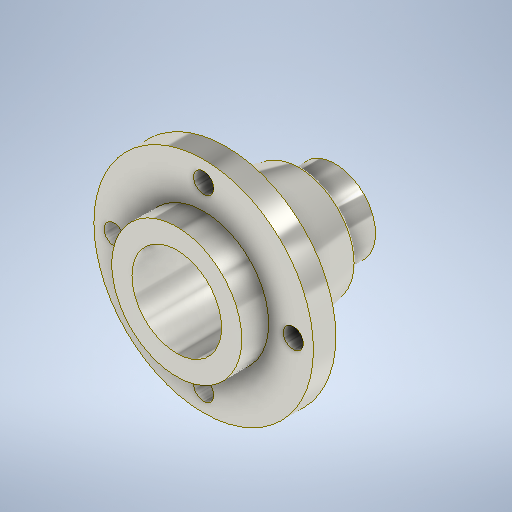
# Autodesk Inventor part: pokrywa
Saved by Autodesk Inventor 2025.2 (Build 292293000, 293)
## iProperties
Created: 2025-03-22
Part Number: pokrywa
Material: Srebro
Document SubType Name: Modeling
Designer: barte
Density: 10.49 g/cm^3
Appearance: Srebro
Author: barte
Autodesk Inventor part; units mm, degrees
ref_plane "YZ Plane" through (0, 0, 0) normal (1, 0, 0) x (0, 1, 0)
ref_plane "XZ Plane" through (0, 0, 0) normal (0, 1, 0) x (-1, 0, 0)
ref_plane "XY Plane" through (0, 0, 0) normal (0, 0, 1) x (1, 0, 0)
sketch "Szkic1" plane through (0, 0, 0) normal (0, 1, 0) x (-1, 0, 0)
  line L0 (34.3124, 12.606) -> (49, 12.606)
  line L1 (0, 12.606) -> (0, -21.394)
  line L2 (20, -21.394) -> (22.7076, -21.394)
  line L3 (49, 12.606) -> (32.75, 12.606)
  line L4 (32.3719, 11.09) -> (24.6481, -19.878)
  arc A0 (34.3124, 12.606) -> (32.3719, 11.09) centre (34.3124, 10.606) ccw
  arc A1 (22.7076, -21.394) -> (24.6481, -19.878) centre (22.7076, -19.394) ccw
  line L5 (49, 12.606) -> (49, 22.606)
  line L6 (49, 22.606) -> (0, 22.606)
  line L7 (0, 22.606) -> (0, 12.606)
  line L8 (0, -21.394) -> (18, -21.394)
  line L9 (18, -23.394) -> (18, -36.124)
  line L10 (18, -36.124) -> (0, -36.124)
  line L11 (0, -36.124) -> (0, -21.394)
  arc A2 (20, -21.394) -> (18, -23.394) centre (20, -23.394) ccw
  point P0 (0, 0)
  point P1 (24.27, -21.394)
  dimension "d0" = 49
  dimension "d1" = 34
  dimension "d2" = 24.27
  dimension "d3" = 16.25
  dimension "d4" = 2
  dimension "d5" = 2
  dimension "d6" = 10
  dimension "d7" = 18
  dimension "d8" = 14.73
  dimension "d9" = 2
  constraints: 24 end point, 8 point on line, 6 point on circle, 6 tangent, 3 centre point, 3 perpendicular, 3 vertical, 2 horizontal, 1 collinear
  measures "d0" distance of L1.start L0.end
  measures "d1" distance of L1.start L1.end
  measures "d2" distance of L1.end point (24.27, -21.394)
  measures "d3" distance of L0.end L3.end
  measures "d4" radius of A0
  measures "d5" radius of A1
  measures "d6" distance of L0.end L5.end
  measures "d7" distance of L1.end L8.end
  measures "d8" distance of L8.end L9.end
  measures "d9" radius of A2
revolve "Obrót1" add sketch "Szkic1" angle 360 about axis through (0, 0, 12.606) along (0, 0, -1)
sketch "Szkic4" plane through (0, 0, 22.606) normal (0, 0, 1) x (1, 0, 0)
  circle A0 centre (0, 0) radius 8
  dimension "d16" = 16
  constraints: 1 centre point, 1 coincident
  measures "d16" diameter of A0
sketch "Szkic5" plane through (0, 0, 22.606) normal (0, 0, 1) x (1, 0, 0)
  circle A0 centre (0, 0) radius 40
  circle A1 centre (-40, 0) radius 4.5
  circle A2 centre (0, -40) radius 4.5
  circle A3 centre (40, 0) radius 4.5
  circle A4 centre (0, 40) radius 4.5
  point P0 (-39.7469, -4.4929)
  point P1 (-39.7469, 4.4929)
  dimension "d21" = 80
  dimension "d22" = 9
  dimension "d31" = 9
  dimension "d32" = 9
  dimension "d33" = 9
  constraints: 5 centre point, 4 point on circle, 1 coincident
  measures "d21" diameter of A0
  measures "d22" diameter of A1
  measures "d31" diameter of A2
  measures "d32" diameter of A3
  measures "d33" diameter of A4
extrude "Wyciągnięcie proste3" cut sketch "Szkic5" against normal through all contours A0 A3 | A0 A3 | A4 A0 | A0 A4 | A2 A0 | A0 A2 | A1 A0 | A0 A1
extrude "Wyciągnięcie proste5" cut sketch "Szkic4" against normal blind 60
sketch "Szkic7" plane through (0, 0, 22.606) normal (0, 0, 1) x (1, 0, 0)
  circle A0 centre (0, 0) radius 29
  constraints: 1 centre point, 1 coincident
extrude "Wyciągnięcie proste6" add sketch "Szkic7" along normal blind 12
sketch "Szkic8" plane through (0, 0, 34.606) normal (0, 0, 1) x (1, 0, 0)
  circle A0 centre (0, 0) radius 8 projected
  circle A1 centre (0, 0) radius 20
  constraints: 1 centre point, 1 coincident
extrude "Wyciągnięcie proste7" cut sketch "Szkic8" against normal blind 47 contours A0 | A1
sketch "Szkic9" plane through (0, 0, -12.394) normal (0, 0, 1) x (1, 0, 0)
  circle A0 centre (0, 0) radius 10
  circle A1 centre (0, 0) radius 8
  constraints: 2 centre point, 2 coincident
extrude "Wyciągnięcie proste8" add sketch "Szkic9" along normal blind 7
